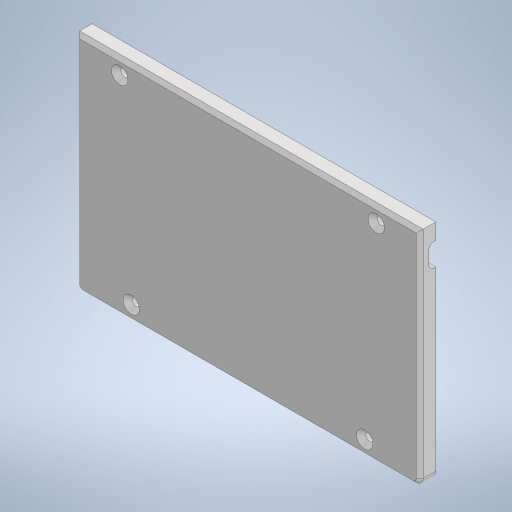
# Autodesk Inventor part: e_box_lid
Saved by Autodesk Inventor 2024.1 (Build 281209000, 209)
## iProperties
Created: 2023-10-22
Part Number: e_box_lid
Material: Generic
Document SubType Name: Modeling
Designer: l1534
Density: 1 g/cm^3
Appearance: Default
Author: l1534
Autodesk Inventor part; units mm, degrees
ref_plane "YZ Plane" through (0, 0, 0) normal (1, 0, 0) x (0, 1, 0)
ref_plane "XZ Plane" through (0, 0, 0) normal (0, 1, 0) x (-1, 0, 0)
ref_plane "XY Plane" through (0, 0, 0) normal (0, 0, 1) x (1, 0, 0)
sketch "Sketch1" plane through (0, 0, 0) normal (0, 0, 1) x (1, 0, 0)
  line L0 (-49.9648, 36.7279) -> (100.0352, 36.7279)
  line L1 (100.0352, 36.7279) -> (100.0352, -60.5221)
  line L2 (100.0352, -60.5221) -> (-49.9648, -60.5221)
  line L3 (-49.9648, -60.5221) -> (-49.9648, 36.7279)
  point P0 (0, 0)
  dimension "d0" = 150
  dimension "d1" = 97.25
  constraints: 8 end point, 2 parallel, 1 horizontal, 1 perpendicular
  measures "d0" distance of L0.start L0.end
  measures "d1" distance of L0.end L1.end
extrude "Extrusion1" add sketch "Sketch1" along normal blind 7
sketch "Sketch2" plane through (0, 0, 0) normal (0, 0, -1) x (-1, 0, 0)
  line L0 (47.4648, -58.0221) -> (-97.5352, -58.0221)
  line L1 (-97.5352, -58.0221) -> (-97.5352, 34.2279)
  line L2 (-97.5352, 34.2279) -> (47.4648, 34.2279)
  line L3 (47.4648, 34.2279) -> (47.4648, -58.0221)
  line L4 (49.9648, -60.5221) -> (-100.0352, -60.5221) projected
  line L5 (-100.0352, -60.5221) -> (-100.0352, 36.7279) projected
  line L6 (49.9648, 36.7279) -> (49.9648, -60.5221) projected
  line L7 (-100.0352, 36.7279) -> (49.9648, 36.7279) projected
  point P0 (0, 0)
  dimension "d4" = 2.5
  dimension "d5" = 2.5
  dimension "d6" = 2.5
  dimension "d7" = 2.5
  constraints: 8 end point, 2 parallel, 1 horizontal, 1 perpendicular
  measures "d4" distance between parallel lines of L4 L0
  measures "d5" distance between parallel lines of L5 L1
  measures "d6" distance between parallel lines of L6 L3
  measures "d7" distance between parallel lines of L7 L2
extrude "Extrusion2" cut sketch "Sketch2" against normal blind 5 contours L0 L1 L2 L3
sketch "Sketch3" plane through (0, 0, 5) normal (0, 0, -1) x (-1, 0, 0)
  line L0 (47.4648, -58.0221) -> (-97.5352, -58.0221) projected
  line L1 (29.9648, -58.0221) -> (21.9648, -58.0221)
  line L2 (21.9648, -58.0221) -> (21.9648, -50.0221)
  line L3 (21.9648, -50.0221) -> (29.9648, -50.0221)
  line L4 (29.9648, -50.0221) -> (29.9648, -58.0221)
  line L5 (-80.0352, -58.0221) -> (-72.0352, -58.0221)
  line L6 (-72.0352, -58.0221) -> (-72.0352, -50.0221)
  line L7 (-72.0352, -50.0221) -> (-80.0352, -50.0221)
  line L8 (-80.0352, -50.0221) -> (-80.0352, -58.0221)
  line L9 (34.9648, 26.2279) -> (26.9648, 26.2279)
  line L10 (26.9648, 26.2279) -> (26.9648, 34.2279)
  line L11 (26.9648, 34.2279) -> (34.9648, 34.2279)
  line L12 (34.9648, 34.2279) -> (34.9648, 26.2279)
  line L13 (-77.0352, 26.2279) -> (-85.0352, 26.2279)
  line L14 (-85.0352, 26.2279) -> (-85.0352, 34.2279)
  line L15 (-85.0352, 34.2279) -> (-77.0352, 34.2279)
  line L16 (-77.0352, 34.2279) -> (-77.0352, 26.2279)
  line L17 (-100.0352, -60.5221) -> (-100.0352, 36.7279) projected
  line L18 (49.9648, 36.7279) -> (49.9648, -60.5221) projected
  line L19 (-100.0352, 36.7279) -> (49.9648, 36.7279) projected
  point P0 (0, 0)
  dimension "d10" = 8
  dimension "d11" = 8
  dimension "d12" = 8
  dimension "d13" = 20
  dimension "d14" = 20
  dimension "d15" = 8
  dimension "d16" = 8
  dimension "d17" = 8
  dimension "d18" = 8
  dimension "d19" = 15
  dimension "d20" = 15
  dimension "d21" = 10.5
  constraints: 32 end point, 8 parallel, 4 horizontal, 4 perpendicular, 4 point on line
  measures "d10" distance of L2.end L3.end
  measures "d11" distance of L1.end L2.end
  measures "d12" distance of L6.end L7.end
  measures "d13" distance between parallel lines of L17 L8
  measures "d14" distance between parallel lines of L18 L4
  measures "d15" distance of L9.end L10.end
  measures "d16" distance of L9.start L9.end
  measures "d17" distance of L13.end L14.end
  measures "d18" distance of L13.start L13.end
  measures "d19" distance between parallel lines of L17 L14
  measures "d20" distance between parallel lines of L18 L12
  measures "d21" distance between parallel lines of L19 L9
extrude "Extrusion3" add sketch "Sketch3" along normal up to surface (5 mm away)
sketch "Sketch4" plane through (0, 0, 0) normal (0, 0, -1) x (-1, 0, 0)
  circle A0 centre (25.9648, -54.0221) radius 1.6
  circle A1 centre (-76.0352, -54.0221) radius 1.6
  line L0 (49.9648, 36.7279) -> (49.9648, -60.5221) projected
  line L1 (49.9648, -60.5221) -> (-100.0352, -60.5221) projected
  line L2 (-100.0352, -60.5221) -> (-100.0352, 36.7279) projected
  circle A2 centre (30.9648, 30.2279) radius 1.6
  circle A3 centre (-81.0352, 30.2279) radius 1.6
  line L3 (-100.0352, 36.7279) -> (49.9648, 36.7279) projected
  point P0 (0, 0)
  dimension "d24" = 3.2
  dimension "d25" = 3.2
  dimension "d26" = 24
  dimension "d27" = 6.5
  dimension "d28" = 24
  dimension "d29" = 6.5
  dimension "d30" = 3.2
  dimension "d31" = 3.2
  dimension "d32" = 19
  dimension "d33" = 6.5
  dimension "d34" = 6.5
  dimension "d35" = 19
  constraints: 4 centre point
  measures "d24" diameter of A1
  measures "d25" diameter of A0
  measures "d26" distance from line of L0 A0.centre
  measures "d27" distance from line of L1 A0.centre
  measures "d28" distance from line of L2 A1.centre
  measures "d29" distance from line of L1 A1.centre
  measures "d30" diameter of A2
  measures "d31" diameter of A3
  measures "d32" distance from line of L2 A3.centre
  measures "d33" distance from line of L3 A3.centre
  measures "d34" distance from line of L3 A2.centre
  measures "d35" distance from line of L0 A2.centre
extrude "Extrusion4" cut sketch "Sketch4" against normal through all contours A0 | A1 | A2 | A3
fillet "Fillet1" radius 3 2 edges at (100.0352, -60.5221, 3.5) (-49.9648, -60.5221, 3.5)
sketch "Sketch5" plane through (100.0352, 36.7279, 7) normal (1, 0, 0) x (0, 0, -1)
  line L0 (7, -17) -> (4, -17)
  line L1 (4, -17) -> (4, -7)
  line L2 (4, -7) -> (7, -7)
  line L3 (7, -7) -> (7, -17)
  line L4 (7, -94.25) -> (7, 0) projected
  line L5 (7, 0) -> (0, 0) projected
  point P0 (7, -36.7279)
  dimension "d39" = 3
  dimension "d40" = 7
  dimension "d41" = 10
  constraints: 8 end point, 2 parallel, 1 collinear, 1 horizontal, 1 perpendicular
  measures "d39" distance of L1.end L2.end
  measures "d40" distance between parallel lines of L5 L2
  measures "d41" distance of L0.end L1.end
extrude "Extrusion5" cut sketch "Sketch5" against normal up to surface (2.5 mm away)
fillet "Fillet2" radius 2 2 edges at (98.7852, 29.7279, 3) (98.7852, 19.7279, 3)
sketch "Sketch6" plane through (-49.9648, 36.7279, 0) normal (-1, 0, 0) x (0, 0, 1)
  line L0 (0, -2.5) -> (0, -94.75) projected
  line L1 (0, -7) -> (3, -7)
  line L2 (3, -7) -> (3, -17)
  line L3 (3, -17) -> (0, -17)
  line L4 (0, -17) -> (0, -7)
  line L5 (0, 0) -> (7, 0) projected
  point P0 (0, -36.7279)
  point P1 (0, -17)
  dimension "d45" = 3
  dimension "d46" = 10
  dimension "d47" = 7
  constraints: 8 end point, 2 parallel, 1 horizontal, 1 perpendicular, 1 point on line
  measures "d45" distance of L2.end L3.end
  measures "d46" distance of L1.end L2.end
  measures "d47" distance between parallel lines of L5 L1
extrude "Extrusion6" cut sketch "Sketch6" against normal up to surface (2.5 mm away)
fillet "Fillet3" radius 2 2 edges at (-48.7148, 29.7279, 3) (-48.7148, 19.7279, 3)
chamfer "Chamfer1" distance 1.5 angle 45 6 edges at (25.0352, 36.7279, 7) (-49.9648, -10.3971, 7) (-49.0861, -59.6434, 7) (25.0352, -60.5221, 7) (99.1566, -59.6434, 7) (100.0352, -10.3971, 7)
sketch "Sketch7" plane through (-46.9648, -60.5221, 0) normal (0, -1, 0) x (1, 0, 0)
  line L0 (147, 0) -> (-3, 0) projected
  line L1 (133.5, 0) -> (144.5, 0)
  line L2 (144.5, 0) -> (144.5, 5)
  line L3 (144.5, 5) -> (133.5, 5)
  line L4 (133.5, 5) -> (133.5, 0)
  line L5 (147, 0) -> (147, 5.5) projected
  point P0 (46.9648, 0)
  dimension "d54" = 5
  dimension "d55" = 11
  dimension "d56" = 2.5
  constraints: 8 end point, 2 parallel, 1 horizontal, 1 perpendicular, 1 point on line
  measures "d54" distance of L1.end L2.end
  measures "d55" distance of L2.end L3.end
  measures "d56" distance between parallel lines of L5 L2
extrude "Extrusion7" cut sketch "Sketch7" against normal up to surface (2.5 mm away)
chamfer "Chamfer2" distance 2 angle 45 4 edges at (-29.3648, 30.2279, 7) (-24.3648, -54.0221, 7) (77.6352, -54.0221, 7) (82.6352, 30.2279, 7)
body "Solid1"
